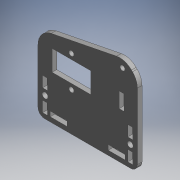
# Autodesk Inventor part: Part11
Saved by Autodesk Inventor 2019.2 (Build 232265000, 265)
## iProperties
Part Number: Part11
Material: Generic
Document SubType Name: Modeling
Designer: richard.girt
Mass: 6.87981 g
Surface Area: 62.6223 cm^2
Volume: 6.87981 cm^3
Density: 1 g/cm^3
Appearance: Default
Author: richard.girt
Autodesk Inventor part; units mm, degrees
ref_plane "YZ Plane" through (0, 0, 0) normal (1, 0, 0) x (0, 1, 0)
ref_plane "XZ Plane" through (0, 0, 0) normal (0, 1, 0) x (-1, 0, 0)
ref_plane "XY Plane" through (0, 0, 0) normal (0, 0, 1) x (1, 0, 0)
sketch "Sketch1" plane through (0, 0, 0) normal (0, 0, 1) x (1, 0, 0)
  line L0 (-30, 0) -> (30, 0)
  line L1 (30, 0) -> (30, 48.0711)
  line L2 (-30, 43.214) -> (-30, 0)
  line L3 (-21.5, 39) -> (1.9, 39)
  line L4 (1.9, 39) -> (1.9, 26.5)
  line L5 (1.9, 26.5) -> (-21.5, 26.5)
  line L6 (-21.5, 26.5) -> (-21.5, 39)
  line L7 (-22.6, 5.7) -> (-12.4, 5.7)
  line L8 (-12.4, 5.7) -> (-12.4, 2.7)
  line L9 (-12.4, 2.7) -> (-22.6, 2.7)
  line L10 (-22.6, 2.7) -> (-22.6, 5.7)
  line L11 (19, 37) -> (22, 37)
  line L12 (22, 37) -> (22, 27.75)
  line L13 (22, 27.75) -> (19, 27.75)
  line L14 (19, 27.75) -> (19, 37)
  line L15 (12.4, 5.7) -> (22.6, 5.7)
  line L16 (22.6, 5.7) -> (22.6, 2.7)
  line L17 (22.6, 2.7) -> (12.4, 2.7)
  line L18 (12.4, 2.7) -> (12.4, 5.7)
  line L19 (-30, 43.214) -> (22.5695, 55.5016)
  line L20 (22.5695, 55.5016) -> (30, 48.0711)
  line L21 (-12.4, 4.2) -> (12.4, 4.2)
  point P0 (0, 0)
  point P1 (0, 0)
  point P2 (21, 50)
  point P3 (0, 4.2)
  dimension "d0" = 60
  dimension "d1" = 43.214
  dimension "d2" = 23.4
  dimension "d3" = 12.5
  dimension "d4" = 8.5
  dimension "d6" = 3
  dimension "d8" = 8
  dimension "d9" = 9.25
  dimension "d10" = 10.2
  dimension "d11" = 10.2
  dimension "d14" = 2.7
  dimension "d33" = 37
  dimension "d34" = 26.5
  dimension "d35" = 50
  dimension "d36" = 9
  dimension "d38" = 5
  dimension "d39" = 5
  dimension "d40" = 45
  dimension "d41" = 24.8
  constraints: 44 end point, 9 parallel, 6 perpendicular, 5 horizontal, 4 midpoint, 2 collinear, 1 coincident, 1 vertical alignment
  measures "d0" distance of L0.start L0.end
  measures "d1" distance of L2.start L0.start
  measures "d2" distance of L3.start L3.end
  measures "d3" distance of L3.end L4.end
  measures "d4" distance between parallel lines of L2 L6
  measures "d6" distance of L11.start L11.end
  measures "d8" distance between parallel lines of L1 L12
  measures "d9" distance of L11.end L12.end
  measures "d10" distance of L8.end L9.end
  measures "d11" distance of L16.end L17.end
  measures "d14" distance between parallel lines of L17 L0
  measures "d33" distance between parallel lines of L0 L11
  measures "d34" distance between parallel lines of L0 L5
  measures "d35" distance from line of L0 point (21, 50)
  measures "d36" distance from line of L1 point (21, 50)
  measures "d38" distance from line of L19 point (21, 50)
  measures "d39" distance from line of L20 point (21, 50)
  measures "d40" angle of L1 L20
  measures "d41" distance of L21.start L21.end
extrude "Extrusion1" add sketch "Sketch1" along normal blind 2.8
sketch "Sketch2" plane through (0, 0, 2.8) normal (0, 0, 1) x (1, 0, 0)
  line L0 (30, 0) -> (30, 48.0711) construction
  line L1 (-30, 43.214) -> (-30, 0) construction
  line L2 (-27.3, 21.9) -> (-24.3, 21.9)
  line L3 (-24.3, 21.9) -> (-24.3, 15.7)
  line L4 (-24.3, 15.7) -> (-27.3, 15.7)
  line L5 (-27.3, 15.7) -> (-27.3, 21.9)
  line L6 (-27.3, 8.9) -> (-24.3, 8.9)
  line L7 (-24.3, 8.9) -> (-24.3, 2.7)
  line L8 (-24.3, 2.7) -> (-27.3, 2.7)
  line L9 (-27.3, 2.7) -> (-27.3, 8.9)
  line L10 (24.3, 2.7) -> (27.3, 2.7)
  line L11 (27.3, 2.7) -> (27.3, 8.9)
  line L12 (27.3, 8.9) -> (24.3, 8.9)
  line L13 (24.3, 8.9) -> (24.3, 2.7)
  line L14 (24.3, 15.7) -> (27.3, 15.7)
  line L15 (27.3, 15.7) -> (27.3, 21.9)
  line L16 (27.3, 21.9) -> (24.3, 21.9)
  line L17 (24.3, 21.9) -> (24.3, 15.7)
  line L18 (-30, 0) -> (30, 0) construction
  line L19 (25.8, 15.7) -> (25.8, 8.9) construction
  line L20 (-25.8, 15.7) -> (-25.8, 8.9)
  point P0 (0, 0)
  point P1 (25.8, 12.3)
  point P2 (-25.8, 12.3)
  dimension "d19" = 2.7
  dimension "d20" = 2.7
  dimension "d49" = 12.3
  dimension "d50" = 3
  dimension "d51" = 12.3
  dimension "d52" = 6.2
  dimension "d53" = 19.2
  constraints: 36 end point, 8 parallel, 6 midpoint, 5 equal length, 4 perpendicular, 4 point on line, 3 horizontal, 1 collinear
  measures "d19" distance between parallel lines of L1 L9
  measures "d20" distance between parallel lines of L11 L0
  measures "d49" distance from line of point (25.8, 12.3) L18
  measures "d50" distance of L10.start L10.end
  measures "d51" distance from line of point (-25.8, 12.3) L18
  measures "d52" distance of L8.end L6.start
  measures "d53" distance between parallel lines of L2 L8
extrude "Extrusion2" cut sketch "Sketch2" against normal blind 2.8
sketch "Sketch3" plane through (0, 0, 2.8) normal (0, 0, 1) x (1, 0, 0)
  line L0 (24.3, 8.9) -> (27.3, 8.9) construction
  line L1 (-24.3, 15.7) -> (-27.3, 15.7) construction
  line L2 (-27.3, 8.9) -> (-24.3, 8.9) construction
  line L3 (27.3, 15.7) -> (24.3, 15.7) construction
  line L4 (1.9, 39) -> (1.9, 26.5) construction
  line L5 (-21.5, 39) -> (1.9, 39) construction
  line L6 (-9.8, 42.25) -> (-9.8, 32.75)
  line L7 (-9.8, 32.75) -> (-9.8, 23.25)
  line L8 (-25.8, 15.7) -> (-25.8, 8.9)
  line L9 (25.8, 15.7) -> (25.8, 8.9)
  point P0 (0, 0)
  point P1 (-25.8, 12.3)
  point P2 (25.8, 12.3)
  point P3 (1.9, 32.75)
  point P4 (-9.8, 39)
  point P5 (21, 50)
  dimension "d23" = 19
  constraints: 8 end point, 8 midpoint, 2 coincident, 2 point on line, 1 collinear, 1 horizontal alignment, 1 vertical
  measures "d23" distance of L7.end L6.start
hole "Hole1" at (-25.8, 12.3, 2.8) at (25.8, 12.3, 2.8) at (-9.8, 23.25, 2.8) at (-9.8, 42.25, 2.8) at (21, 50, 2.8) direction (0, 0, -1) diameter 3 end through all
sketch "Sketch4" plane through (0, 0, 2.8) normal (0, 0, 1) x (1, 0, 0)
  circle A0 centre (25.8, 12.3) radius 1.5 construction
  circle A1 centre (-25.8, 12.3) radius 1.5 construction
  point P0 (0, 0)
  constraints: 2 coincident
hole "Hole2" at (-25.8, 12.3, 2.8) at (25.8, 12.3, 2.8) direction (0, 0, -1) diameter 3.5 end through all
fillet "Fillet1" radius 4 2 edges at (30, 0, 1.4) (-30, 0, 1.4)
fillet "Fillet2" radius 10 3 edges at (-30, 43.214, 1.4) (30, 48.0711, 1.4) (22.5695, 55.5016, 1.4)
equation "\"d11\" = d10"
body "Solid1"
